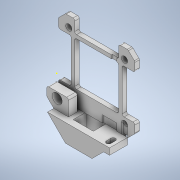
# Autodesk Inventor part: mechaduino_mount3
Saved by Autodesk Inventor 2020.3 (Build 243373000, 373)
## iProperties
Created: 2020-12-19
Part Number: mechaduino_mount3
Material: Generic
Document SubType Name: Modeling
Designer: Martijn
Density: 1 g/cm^3
Appearance: Default
Author: Martijn
Autodesk Inventor part; units mm, degrees
ref_plane "YZ Plane" through (0, 0, 0) normal (1, 0, 0) x (0, 1, 0)
ref_plane "XZ Plane" through (0, 0, 0) normal (0, 1, 0) x (-1, 0, 0)
ref_plane "XY Plane" through (0, 0, 0) normal (0, 0, 1) x (1, 0, 0)
sketch "Sketch1" plane through (0, 0, 0) normal (0, 0, 1) x (1, 0, 0)
  line L0 (0, 0) -> (0, 12.2)
  line L1 (0, 12.2) -> (0, 12.2)
  line L2 (0, 12.2) -> (0, 12.2)
  line L3 (0, 12.2) -> (12.2, 12.2)
  line L4 (12.2, 12.2) -> (12.2, 14.2)
  line L5 (-2, 0) -> (0, 0)
  line L6 (12.2, 14.2) -> (0, 14.2)
  line L7 (0, 14.2) -> (0, 21.2)
  line L8 (0, 21.2) -> (-5.1816, 21.2)
  line L9 (-2, 0) -> (-2, 12.2)
  line L10 (-2, 12.2) -> (-9, 12.2)
  line L11 (-9, 12.2) -> (-9, 17.3816)
  line L12 (-9, 17.3816) -> (-5.1816, 21.2)
  dimension "d0" = 2
  dimension "d1" = 2
  dimension "d19" = 135
  dimension "d20" = 21.2
  dimension "d21" = 21.2
  dimension "d22" = 5.4
  dimension "d23" = 9
  dimension "d24" = 9
  constraints: 26 end point, 8 perpendicular, 4 collinear, 2 vertical, 1 horizontal
  measures "d0" distance of L5.start L0.start
  measures "d1" distance of L3.end L4.end
  measures "d19" angle of L12 L8
  measures "d20" distance between parallel lines of L4 L11
  measures "d21" distance between parallel lines of L5 L8
  measures "d22" distance of L11.end L8.end
  measures "d23" distance between parallel lines of L1 L8
  measures "d24" distance between parallel lines of L11 L2
extrude "Extrusion1" add sketch "Sketch1" along normal blind 2.5
sketch "Sketch2" plane through (0, 0, 2.5) normal (0, 0, 1) x (1, 0, 0)
  circle A0 centre (-3.3, 15.5) radius 1.7
  line L0 (-2, 0) -> (0, 0) projected
  line L1 (12.2, 12.2) -> (12.2, 14.2) projected
  dimension "d9" = 15.5
  dimension "d10" = 15.5
  dimension "d11" = 3.4
  constraints: 1 centre point
  measures "d9" distance from line of L0 A0.centre
  measures "d10" distance from line of L1 A0.centre
  measures "d11" diameter of A0
extrude "Extrusion2" cut sketch "Sketch2" against normal blind 10
fillet "Fillet3" radius 1 7 edges at (0, 12.2, 1.25) (-2, 12.2, 1.25) (0, 14.2, 1.25) (-9, 12.2, 1.25) (0, 21.2, 1.25) (-5.1816, 21.2, 1.25) (-9, 17.3816, 1.25)
mirror "Mirror3" about plane through (12.2, 12.2, 0) normal (1, 0, 0)
mirror "Mirror4" about plane through (26.4, 0, 0) normal (0, -1, 0)
sketch "Sketch4" plane through (0, 0, 2.5) normal (0, 0, 1) x (1, 0, 0)
  line L0 (1, 14.2) -> (23.4, 14.2) projected
  line L1 (1, 12.2) -> (23.4, 12.2) projected
  line L2 (23.4, 14.2) -> (20.4, 14.2)
  line L3 (20.4, 14.2) -> (20.4, 12.2)
  line L4 (20.4, 12.2) -> (23.4, 12.2)
  line L5 (23.4, 12.2) -> (23.4, 14.2)
  line L6 (33.4, 16.9674) -> (33.4, 13.2) projected
  point P0 (0, 0)
  dimension "d26" = 10
  dimension "d27" = 3
  constraints: 8 end point, 2 parallel, 2 point on line, 1 horizontal, 1 perpendicular
  measures "d26" distance between parallel lines of L6 L5
  measures "d27" distance between parallel lines of L3 L5
extrude "Extrusion3" cut sketch "Sketch4" against normal blind 0.5
sketch "Sketch5" plane through (0, 0, 2.5) normal (0, 0, 1) x (1, 0, 0)
  line L0 (24.4, -15.2) -> (24.4, -20.2) projected
  line L1 (26.0118, -15.7) -> (29.3882, -15.7)
  line L2 (29.3882, -15.7) -> (29.3882, -21.2)
  line L3 (29.3882, -21.2) -> (26.0118, -21.2)
  line L4 (26.0118, -21.2) -> (26.0118, -15.7)
  circle A0 centre (27.7, -15.5) radius 1.7 projected
  line L5 (25.4, -21.2) -> (29.1674, -21.2) projected
  point P0 (0, 0)
  dimension "d30" = 5.5
  constraints: 8 end point, 2 parallel, 2 point on circle, 1 collinear, 1 horizontal, 1 perpendicular
  measures "d30" distance between parallel lines of L1 L3
extrude "Extrusion4" cut sketch "Sketch5" against normal blind 1 contours A0 L2 L3 L4
sketch "Sketch6" plane through (0, 0, 0) normal (0, 0, -1) x (-1, 0, 0)
  line L0 (-25.4, -21.2) -> (-29.1674, -21.2) projected
  line L1 (1, -14.2) -> (-25.4, -14.2)
  line L2 (-25.4, -14.2) -> (-25.4, -21.2)
  line L3 (-25.4, -21.2) -> (1, -21.2)
  line L4 (1, -21.2) -> (1, -14.2)
  line L5 (-1, -14.2) -> (-23.4, -14.2) projected
  point P0 (0, 0)
  constraints: 8 end point, 2 parallel, 1 coincident, 1 collinear, 1 horizontal, 1 perpendicular
extrude "Extrusion5" add sketch "Sketch6" against normal up to surface (2.5 mm away)
sketch "Sketch7" plane through (0, 0, 2.5) normal (0, 0, 1) x (1, 0, 0)
  line L0 (29.1674, -21.2) -> (-4.7674, -21.2) projected
  line L1 (15.4, -17.2) -> (23.4, -17.2)
  line L2 (23.4, -17.2) -> (23.4, -21.2)
  line L3 (23.4, -21.2) -> (15.4, -21.2)
  line L4 (15.4, -21.2) -> (15.4, -17.2)
  line L5 (33.4, -16.9674) -> (33.4, -13.2) projected
  point P0 (0, 0)
  dimension "d36" = 10
  dimension "d37" = 4
  dimension "d38" = 8
  constraints: 8 end point, 2 parallel, 1 horizontal, 1 perpendicular, 1 point on line
  measures "d36" distance between parallel lines of L5 L2
  measures "d37" distance between parallel lines of L0 L1
  measures "d38" distance between parallel lines of L2 L4
extrude "Extrusion6" cut sketch "Sketch7" against normal blind 0.5
sketch "Sketch11" plane through (0, 0, 2.5) normal (0, 0, 1) x (1, 0, 0)
  arc A0 (-8, -12.2) -> (-9, -13.2) centre (-8, -13.2) ccw projected
  arc A1 (-8, -12.2) -> (-9, -13.2) centre (-8, -13.2) ccw
  line L0 (-8, -12.2) -> (2, -12.2)
  line L1 (-8, -12.2) -> (-3, -12.2) projected
  arc A2 (3, -13.2) -> (2, -12.2) centre (2, -13.2) ccw
  line L2 (3, -13.2) -> (3, -21.2)
  line L3 (4.8184, -31.2) -> (-5.1816, -21.2)
  line L4 (-5.4745, -20.9071) -> (-8.7071, -17.6745) projected
  line L5 (-5.1816, -21.2) -> (-8.7071, -17.6745)
  arc A3 (-9, -16.9674) -> (-8.7071, -17.6745) centre (-8, -16.9674) ccw
  line L6 (-9, -16.9674) -> (-9, -13.2)
  arc A4 (-9, -16.9674) -> (-8.7071, -17.6745) centre (-8, -16.9674) ccw projected
  line L7 (29.8745, -20.9071) -> (33.1071, -17.6745) projected
  line L8 (3, -21.2) -> (5.6, -21.2)
  line L9 (5.6, -21.2) -> (5.6, -31.2)
  line L10 (5.6, -31.2) -> (4.8184, -31.2)
  line L11 (19.5816, -31.2) -> (16.8, -31.2)
  circle A5 centre (-3.3, -15.5) radius 1.7 projected
  circle A6 centre (-3.3, -15.5) radius 1.7
  circle A7 centre (-3.3, -15.5) radius 1.7 projected
  line L12 (26.0118, -21.2) -> (26.0118, -24.7698)
  line L13 (26.0118, -24.7698) -> (19.5816, -31.2)
  line L14 (26.0118, -24.7698) -> (29.5816, -21.2)
  line L15 (26.0118, -21.2) -> (23.4, -21.2) projected
  line L16 (26.0118, -21.2) -> (16.8, -21.2)
  line L17 (23.4, -21.2) -> (15.4, -21.2) projected
  line L18 (16.8, -31.2) -> (16.8, -21.2)
  line L19 (15.4, -21.2) -> (-4.7674, -21.2) projected
  line L20 (33.4, -16.9674) -> (33.4, -13.2) projected
  point P0 (0, 0)
  dimension "d53" = 12
  dimension "d54" = 1
  dimension "d60" = 10
  dimension "d81" = 45
  dimension "d83" = 45
  dimension "d92" = 14.6
  dimension "d93" = 16.6
  dimension "d94" = 11.2
  constraints: 28 end point, 6 point on circle, 5 collinear, 4 centre point, 4 point on line, 3 concentric, 3 vertical, 2 coincident, 2 perpendicular, 2 tangent, 1 horizontal, 1 parallel
  measures "d53" distance between parallel lines of L6 L2
  measures "d54" radius of A2
  measures "d60" distance between parallel lines of L10 L8
  measures "d81" angle of L15 L14
  measures "d83" angle of L3 L8
  measures "d92" distance between parallel lines of L6 L9
  measures "d93" distance between parallel lines of L20 L18
  measures "d94" distance between parallel lines of L18 L9
extrude "Extrusion10" add sketch "Sketch11" along normal blind 6.5
sketch "Sketch12" plane through (0, 0, 9) normal (0, 0, 1) x (1, 0, 0)
  line L0 (-8.7071, -17.6745) -> (4.8184, -31.2) projected
  arc A0 (29.1674, -21.2) -> (29.3882, -21.1753) centre (29.1674, -20.2) ccw projected
  line L1 (4.8184, -31.2) -> (5.6, -31.2) projected
  line L2 (19.5816, -31.2) -> (4.8184, -31.2)
  line L3 (4.8184, -31.2) -> (-5.1816, -21.2)
  line L4 (26.0118, -21.2) -> (16.8, -21.2) projected
  line L5 (-5.1816, -21.2) -> (26.0118, -21.2)
  line L6 (26.0118, -21.2) -> (26.0118, -24.7698)
  line L7 (16.8, -31.2) -> (19.5816, -31.2) projected
  line L8 (26.0118, -24.7698) -> (19.5816, -31.2)
  point P0 (0, 0)
  constraints: 10 end point, 1 collinear, 1 horizontal, 1 perpendicular
extrude "Extrusion11" add sketch "Sketch12" along normal blind 3.5
sketch "Sketch13" plane through (0, 0, 2.5) normal (0, 0, -1) x (-1, 0, 0)
  line L0 (-4.8184, -31.2) -> (-5.6, -31.2) projected
  line L1 (-4.8184, -31.2) -> (-19.5816, -31.2)
  line L2 (6.6816, -19.7) -> (5.1816, -21.2)
  line L3 (5.4745, -20.9071) -> (5.1816, -21.2) projected
  line L4 (5.1816, -21.2) -> (-4.8184, -31.2)
  line L5 (-5.6, -21.2) -> (-3, -21.2) projected
  line L6 (-3, -21.2) -> (-3, -19.7)
  line L7 (-3, -19.7) -> (6.6816, -19.7)
  line L8 (-26.0118, -24.7698) -> (-26.0118, -21.2) projected
  line L9 (-26.0118, -24.7698) -> (-26.0118, -21.2)
  line L10 (-26.0118, -21.2) -> (-3, -21.2)
  line L11 (-3, -21.2) -> (4.7674, -21.2) projected
  line L12 (5.4745, -20.9071) -> (8.7071, -17.6745) projected
  line L13 (-26.0118, -27.1668) -> (-26.0118, -21.2) projected
  line L14 (-16.8, -31.2) -> (-19.5816, -31.2) projected
  line L15 (-26.0118, -24.7698) -> (-19.5816, -31.2)
  point P0 (0, 0)
  dimension "d84" = 1.5
  constraints: 16 end point, 3 point on line, 1 horizontal, 1 perpendicular, 1 vertical
  measures "d84" distance between parallel lines of L7 L5
extrude "Extrusion12" add sketch "Sketch13" along normal up to surface (2.5 mm away)
sketch "Sketch16" plane through (0, 0, 2.5) normal (0, 0, 1) x (1, 0, 0)
  line L0 (5.6, -21.2) -> (3, -21.2) projected
  line L1 (5.6, -21.2) -> (16.8, -21.2)
  line L2 (16.8, -21.2) -> (16.8, -31.2)
  line L3 (16.8, -31.2) -> (5.6, -31.2)
  line L4 (5.6, -31.2) -> (5.6, -21.2)
  line L5 (16.8, -21.2) -> (16.8, -31.2) projected
  line L6 (4.8184, -31.2) -> (19.5816, -31.2) projected
  point P0 (0, 0)
  constraints: 8 end point, 2 collinear, 2 parallel, 1 horizontal, 1 perpendicular
extrude "Extrusion13" cut sketch "Sketch16" against normal blind 1
sketch "Sketch18" plane through (0, 0, 9) normal (0, 0, 1) x (1, 0, 0)
  circle A0 centre (-3.3, -15.5) radius 1.7 projected
  circle A1 centre (-3.3, -15.5) radius 2.75
  point P0 (0, 0)
  dimension "d73" = 5.5
  constraints: 1 centre point, 1 coincident
  measures "d73" diameter of A1
extrude "Extrusion15" cut sketch "Sketch18" against normal up to surface (6.5 mm away)
sketch "Sketch19" plane through (-8, -12.2, 0) normal (0, 1, 0) x (1, 0, 0)
  line L0 (-1, -2.5) -> (-1, 0) projected
  line L1 (11, -4.2) -> (-1, -4.2)
  line L2 (-1, -4.2) -> (-1, -2.5)
  line L3 (-1, -2.5) -> (11, -2.5)
  line L4 (11, -2.5) -> (11, -4.2)
  point P0 (8, 0)
  dimension "d76" = 1.7
  constraints: 8 end point, 2 parallel, 1 horizontal, 1 perpendicular
  measures "d76" distance of L3.end L1.start
extrude "Extrusion16" cut sketch "Sketch19" against normal up to surface (9 mm away)
sketch "Sketch23" plane through (26.0118, -21.2, 1.5) normal (1, 0, 0) x (0, 0, -1)
  point P0 (1.5, 21.2)
sketch "Sketch24" plane through (0, 0, 12.5) normal (0, 0, 1) x (1, 0, 0)
  point P0 (0, 0)
sketch "Sketch25" plane through (26.0118, -21.2, 1.5) normal (1, 0, 0) x (0, 0, -1)
  line L0 (-1, 4) -> (-1, 0) projected
  line L1 (-11, -3.5698) -> (-11, 0) projected
  line L2 (-1, 0) -> (-11, 0)
  line L3 (-11, 0) -> (-11, -3.5698)
  line L4 (-11, -3.5698) -> (-1, -3.5698)
  line L5 (-1, -3.5698) -> (-1, 0)
  point P0 (1.5, 21.2)
  constraints: 8 end point, 2 parallel, 1 horizontal, 1 perpendicular
extrude "Extrusion18" add sketch "Sketch25" along normal blind 3.3
sketch "Sketch26" plane through (-5.1816, -21.2, 9) normal (0, 1, 0) x (1, 0, 0)
  arc A0 (30.2434, -1) -> (32.7434, -1) centre (31.4934, -1) ccw
  line L0 (32.7434, -1) -> (32.7434, 1.5)
  line L1 (30.2434, -1) -> (30.2434, 1.5)
  arc A1 (32.7434, 1.5) -> (30.2434, 1.5) centre (31.4934, 1.5) ccw
  line L2 (34.4934, 6.5) -> (34.4934, -3.5) projected
  line L3 (0, -3.5) -> (34.4934, -3.5) projected
  point P0 (5.1816, 9)
  dimension "d97" = 2.5
  dimension "d98" = 3
  dimension "d99" = 2.5
  dimension "d100" = 2.5
  constraints: 4 end point, 4 point on circle, 4 tangent, 2 centre point, 2 vertical
  measures "d97" distance of L1.start L1.end
  measures "d98" distance from line of L2 A0.centre
  measures "d99" distance between parallel lines of L1 L0
  measures "d100" distance from line of L3 A0.centre
extrude "Extrusion19" cut sketch "Sketch26" against normal blind 10
body "Solid1"
